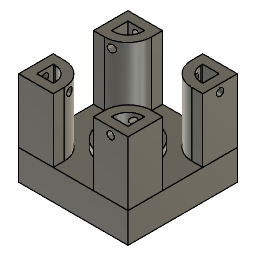
robot (Autodesk Fusion 360 archive; units mm, degrees)
design "pince_v01_structure"
part number: 2026-02-12-14-10-12-234
Autodesk Fusion 360 part; units mm, degrees
(part 1 of 2)
sketch "Esquisse1" plane through (0, 0, 0) normal (0, 0, 1) x (1, 0, 0)
  line L0 (30, 30) -> (-30, 30)
  line L1 (-30, 30) -> (-30, -30)
  line L2 (-30, -30) -> (30, -30)
  line L3 (30, -30) -> (30, 30)
  constraint horizontal L0
  constraint vertical L1
  constraint horizontal L2
  constraint vertical L3
extrude "Extrusion1" add sketch "Esquisse1" along normal blind 5 makes body 1
sketch "Esquisse3" plane through (0, 0, 5) normal (0, 0, 1) x (-1, 0, 0)
  line L0 (-30, 30) -> (-30, -30)
  line L1 (-30, -30) -> (30, -30)
  line L2 (30, -30) -> (30, 30)
  line L3 (30, 30) -> (-30, 30)
  circle A0 centre (0, 0) radius 3.5
  circle A1 centre (0, 0) radius 15
  dimension "d12" = 7
  dimension "d15" = 30
  constraint coincident A0.centre A1.centre
  measures "d12" diameter of A0
  measures "d15" diameter of A1
extrude "Extrusion2" add sketch "Esquisse3" along normal blind 4 contours A1 bodies 1
sketch "Esquisse4" plane through (0, 0, 5) normal (0, 0, 1) x (-1, 0, 0)
  line L0 (-30, 30) -> (-30, -30)
  line L1 (-30, -30) -> (30, -30)
  line L2 (30, -30) -> (30, 30)
  line L3 (30, 30) -> (-30, 30)
  circle A0 centre (0, 0) radius 15
  arc A1 (-24, 11) -> (-11, 24) centre (-24, 24) ccw
  line L4 (-11, 24) -> (-30, 24)
  line L5 (-30, 24) -> (-30, 30)
  line L6 (-30, 30) -> (-11, 30)
  line L7 (-11, 30) -> (-11, 24)
  line L8 (-30, 30) -> (-24, 30)
  line L9 (-24, 30) -> (-24, 11)
  line L10 (-24, 11) -> (-30, 11)
  line L11 (-30, 11) -> (-30, 30)
  constraint horizontal L4
  constraint vertical L5
  constraint horizontal L6
  constraint vertical L7
  constraint coincident L0.start L3.end
  constraint horizontal L8
  constraint vertical L9
  constraint horizontal L10
  constraint vertical L11
extrude "Extrusion3" add sketch "Esquisse4" along normal up to surface (70 mm away) contours L0 L3 L4 L5 L6 L8 L9 L11 | L0 L4 L9 L10 L11 | L3 L4 L6 L7 L9 | A1 L4 L9 bodies 1
sketch "Esquisse5" plane through (0, 0, 0) normal (0, 1, 0) x (1, 0, 0)
  line L0 (-30, 0) -> (30, 0)
  line L1 (30, 0) -> (30, 9.0556)
  line L2 (30, 19.372) -> (-30, 19.372)
  line L3 (-30, 9.0556) -> (-30, 0)
  circle A0 centre (0, 36) radius 34.3
  arc A1 (-25.7143, 10.8052) -> (25.7143, 10.8052) centre (0, 36) ccw
  arc A2 (-25.7143, 10.8052) -> (-30, 9.0556) centre (-27.5, 9.0556) ccw
  arc A3 (30, 9.0556) -> (25.7143, 10.8052) centre (27.5, 9.0556) ccw
  line L4 (-30, 7.5) -> (-27.5, 7.5)
  line L5 (-27.5, 7.5) -> (-27.5, 11.5556)
  line L6 (-27.5, 11.5556) -> (-30, 11.5556)
  line L7 (-30, 11.5556) -> (-30, 7.5)
  point P0 (-30, 0)
  dimension "d80" = 36
  dimension "d81" = 2.5
  dimension "d82" = 2.5
  dimension "d83" = 2.5
  constraint horizontal L0
  constraint vertical L1
  constraint horizontal L2
  constraint vertical L3
  constraint coincident L2.start A0
  constraint coincident P0 L0.start
  constraint coincident A0.centre A1.centre
  constraint tangent A1 A2
  constraint tangent L3 A2
  constraint tangent A1 A3
  constraint tangent L1 A3
  constraint horizontal L4
  constraint vertical L5
  constraint horizontal L6
  constraint vertical L7
  constraint coincident L3 L4.start
  measures "d80" radius of A1
  measures "d81" radius of A2
  measures "d82" radius of A3
  measures "d83" distance of L4.start L4.end
revolve "Révolution2" add sketch "Esquisse5" angle 360 about axis through (0, 0, -205.75) along (0, 0, 1) contours L0 L3 A1 A2 L4 L5 | L3 A2 L4 L5 L7 | A2 L6 L7 bodies 1
extrude "Extrusion4" add 4 faces at (-24.1061, -24.1061, 0) (24.1061, -24.1061, 0) (24.1061, 24.1061, 0) (-24.1061, 24.1061, 0) along direction (0, 0, -1) up to surface end surface through (0, 0, -11.5556) normal (0, 0, -1) offset 0 on bodies 1 bodies 1
extrude "Extrusion5" cut 1 faces at (28, -17.3333, 75) along direction (0, 0, -1) blind 35 on bodies 1 bodies 1
sketch "Esquisse7" plane through (0, 0, 40) normal (0, 0, 1) x (-1, 0, 0)
  line L0 (-30, 11) -> (-24, 11)
  arc A0 (-24, 11) -> (-11, 24) centre (-24, 24) ccw
  line L1 (-11, 24) -> (-11, 30)
  line L2 (-11, 30) -> (-30, 30)
  line L3 (-30, 30) -> (-30, 11)
  line L4 (-16, 24) -> (-16, 25)
  line L5 (-16, 25) -> (-25, 25)
  line L6 (-25, 25) -> (-25, 16)
  line L7 (-25, 16) -> (-24, 16)
  arc A1 (-24, 16) -> (-16, 24) centre (-24, 24) ccw
  dimension "d157" = -5
extrude "Extrusion7" cut sketch "Esquisse7" against normal blind 10 contours L4 L5 L6 L7 A1 bodies 1
pattern_circular "Réseau C2" count 4 over 360 about axis through (0, 0, -205.75) along (0, 0, 1) of bodies 1 makes body 2 at (30, 23.6667, 11.1481) makes body 3 at (-23.6667, 30, 11.1481) makes body 4 at (-30, -23.6667, 11.1481)
sketch "Esquisse8" plane through (0, -30, 0) normal (0, -1, 0) x (1, 0, 0)
  line L0 (30, 40) -> (11, 40)
  line L1 (11, 40) -> (11, 5)
  line L2 (11, 5) -> (-30, 5)
  line L3 (-30, 5) -> (-30, -11.5556)
  line L4 (-30, -11.5556) -> (30, -11.5556)
  line L5 (30, -11.5556) -> (30, 40)
  line L6 (11, 40) -> (30, 40)
  line L7 (30, 40) -> (30, 36)
  line L8 (30, 36) -> (11, 36)
  line L9 (11, 36) -> (11, 40)
  circle A0 centre (20.5, 36) radius 2
  dimension "d3" = 4
  dimension "d4" = 4
  constraint horizontal L6
  constraint vertical L7
  constraint horizontal L8
  constraint vertical L9
  constraint coincident L0.end L1.start
  constraint midpoint L8 A0.centre
  measures "d3" distance of L0.end L8.end
  measures "d4" diameter of A0
extrude "Extrusion8" cut sketch "Esquisse8" against normal up to surface (19 mm away) contours L8 A0 | L8 A0 bodies 1
sketch "Esquisse9" plane through (-30, 0, 0) normal (-1, 0, 0) x (0, -1, 0)
  line L0 (30, 40) -> (11, 40)
  line L1 (11, 40) -> (11, 5)
  line L2 (11, 5) -> (-30, 5)
  line L3 (-30, 5) -> (-30, -11.5556)
  line L4 (-30, -11.5556) -> (30, -11.5556)
  line L5 (30, -11.5556) -> (30, 40)
  line L6 (30, 40) -> (11, 40)
  line L7 (30, 40) -> (30, 36)
  line L8 (30, 36) -> (11, 36)
  line L9 (11, 36) -> (11, 40)
  circle A0 centre (20.5, 36) radius 2
  line L10 (11, 40) -> (30, 40)
  dimension "d7" = 4
  dimension "d8" = 4
  constraint horizontal L10
  constraint vertical L7
  constraint horizontal L8
  constraint vertical L9
  constraint coincident L0.end L1.start
  constraint midpoint A0.centre L8
  measures "d7" distance of L0.end L8.end
  measures "d8" diameter of A0
sketch "Esquisse10" plane through (0, 30, 0) normal (0, 1, 0) x (-1, 0, 0)
  line L0 (30, 40) -> (11, 40)
  line L1 (11, 40) -> (11, 5)
  line L2 (11, 5) -> (-30, 5)
  line L3 (-30, 5) -> (-30, -11.5556)
  line L4 (-30, -11.5556) -> (30, -11.5556)
  line L5 (30, -11.5556) -> (30, 40)
  line L6 (30, 40) -> (11, 40)
  line L7 (30, 40) -> (30, 36)
  line L8 (30, 36) -> (11, 36)
  line L9 (11, 36) -> (11, 40)
  circle A0 centre (20.5, 36) radius 2
  line L10 (11, 40) -> (30, 40)
  dimension "d9" = 4
  dimension "d10" = 4
  constraint horizontal L10
  constraint vertical L7
  constraint horizontal L8
  constraint vertical L9
  constraint coincident L0.end L1.start
  constraint midpoint A0.centre L8
  measures "d9" distance of L0.end L8.end
  measures "d10" diameter of A0
sketch "Esquisse11" plane through (30, 0, 0) normal (1, 0, 0) x (0, 1, 0)
  line L0 (30, 40) -> (11, 40)
  line L1 (11, 40) -> (11, 5)
  line L2 (11, 5) -> (-30, 5)
  line L3 (-30, 5) -> (-30, -11.5556)
  line L4 (-30, -11.5556) -> (30, -11.5556)
  line L5 (30, -11.5556) -> (30, 40)
  line L6 (30, 40) -> (11, 40)
  line L7 (30, 40) -> (30, 36)
  line L8 (30, 36) -> (11, 36)
  line L9 (11, 36) -> (11, 40)
  circle A0 centre (20.5, 36) radius 2
  line L10 (11, 40) -> (30, 40)
  dimension "d11" = 4
  dimension "d16" = 4
  constraint horizontal L10
  constraint vertical L7
  constraint horizontal L8
  constraint vertical L9
  constraint coincident L0.end L1.start
  constraint midpoint A0.centre L8
  measures "d11" distance of L0.end L8.end
  measures "d16" diameter of A0
extrude "Extrusion9" cut sketch "Esquisse9" against normal up to surface (19 mm away) contours L8 A0 | L8 A0 bodies 4
extrude "Extrusion10" cut sketch "Esquisse10" against normal up to surface (19 mm away) contours L8 A0 | L8 A0 bodies 3
extrude "Extrusion11" cut sketch "Esquisse11" against normal up to surface (19 mm away) contours L8 A0 | L8 A0 bodies 2

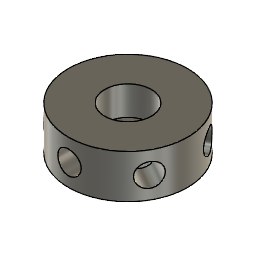
design "encoder_wheel"
part number: 2026-04-24-11-50-52-108
part number: 2026-04-24-11-55-09-590
Autodesk Fusion 360 part; units mm, degrees
sketch "Esquisse1" plane through (0, 0, 0) normal (0, 0, 1) x (1, 0, 0) in component "encoder_wheel"
  line L0 (0, 3.2) -> (-3.2, 0)
  circle A0 centre (0, 0) radius 8.2
  line L1 (-2.5981, -1.5) -> (0, -3)
  line L2 (0, -3) -> (2.5981, -1.5)
  circle A1 centre (0, 0) radius 3.2
  line L3 (-2.5981, 1.5) -> (-2.5981, -1.5)
  line L4 (0, 3) -> (-2.5981, 1.5)
  line L5 (2.5981, -1.5) -> (2.5981, 1.5)
  line L6 (2.5981, 1.5) -> (0, 3)
  dimension "d1" = 6.4
  dimension "d2" = 16.4
  constraint coincident A0.centre A1.centre
  constraint coincident L0.start A1
  constraint coincident L0.end A1
  measures "d1" diameter of A1
  measures "d2" diameter of A0
extrude "Extrusion1" add sketch "Esquisse1" along normal blind 6 in component "encoder_wheel"
extrude "Extrusion2" add sketch "Esquisse1" along normal blind 2 contours L0 A1 L3 L4 | L0 L3 L4 in component "encoder_wheel"
sketch "Esquisse2" plane through (0, 0, 0) normal (0, 1, 0) x (1, 0, 0) in component "encoder_wheel"
  circle A0 through (1.6, -3, -8.2) (-0.8, -1.6144, -8.2) (-0.8, -4.3856, -8.2)
  dimension "d7" = 3.2
extrude "Extrusion3" cut sketch "Esquisse2" along normal blind 3.5 contours A0 in plane through (0, -8.2, 0) normal (0, 1, 0) in component "encoder_wheel"
pattern_circular "Réseau C1" count 6 over 360 about axis through (0, 0, 1.75) along (0, 0, 1) of "Extrusion3" in component "encoder_wheel"
component "encoder_wheel" placed x (1, 0, 0) y (0, 1, 0) z (0, 0, 1) at (0, 0, 0)

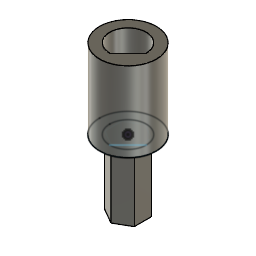
design "wheel-motor_adapter"
part number: 2026-02-08-14-05-17-798
part number: 2026-02-08-22-36-21-611
Autodesk Fusion 360 part; units mm, degrees
sketch "Esquisse1" plane through (0, 0, 0) normal (0, 0, 1) x (1, 0, 0) in component "adaptater"
  line L0 (0, 3) -> (-2.5981, 1.5)
  line L1 (-2.5981, 1.5) -> (-2.5981, -1.5)
  line L2 (-2.5981, -1.5) -> (0, -3)
  line L3 (0, -3) -> (2.5981, -1.5)
  line L4 (2.5981, -1.5) -> (2.5981, 1.5)
  line L5 (2.5981, 1.5) -> (0, 3)
  dimension "d12" = 3
  measures "d12" distance of L0.start origin
extrude "Extrusion1" add sketch "Esquisse1" along normal blind 12 makes body 1 in component "adaptater"
sketch "Esquisse2" plane through (0, 0, 12) normal (0, 0, 1) x (-1, 0, 0) in component "adaptater"
  line L0 (-2.5981, -1.5) -> (0, -3)
  line L1 (0, -3) -> (2.5981, -1.5)
  line L2 (2.5981, -1.5) -> (2.5981, 1.5)
  line L3 (2.5981, 1.5) -> (0, 3)
  line L4 (0, 3) -> (-2.5981, 1.5)
  line L5 (-2.5981, 1.5) -> (-2.5981, -1.5)
  circle A0 centre (0, 0) radius 3.2
  circle A1 centre (0, 0) radius 5
  line L6 (0, 3.2) -> (-3.2, 0)
  dimension "d15" = 6.4
  dimension "d16" = 10
  constraint coincident A0.centre A1.centre
  constraint coincident A0 L6.start
  constraint coincident A0 L6.end
  measures "d15" diameter of A0
  measures "d16" diameter of A1
extrude "Extrusion2" add sketch "Esquisse2" along normal blind 14 bodies 1 makes body 2 in component "adaptater"
extrude "Extrusion3" add sketch "Esquisse2" along normal blind 4 contours L0 L1 L2 L3 L4 L5 L6 | L0 L1 L2 L3 L4 L5 A0 L6 | L4 L5 L6 bodies 1 2 in component "adaptater"
extrude "Extrusion4" add sketch "Esquisse2" along normal blind 4 contours L4 L5 A0 L6 bodies 1 in component "adaptater"
extrude "Extrusion5" add sketch "Esquisse2" along normal blind 14 contours L4 L5 A0 L6 | L4 L5 L6 bodies 1 in component "adaptater"
component "adaptater" placed x (1, 0, 0) y (0, 1, 0) z (0, 0, 1) at (0, 0, 0)

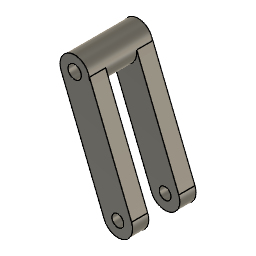
design "pince_v01_second_arm"
part number: 2026-02-12-19-33-38-702
Autodesk Fusion 360 part; units mm, degrees
sketch "Esquisse1" plane through (0, -10.5, 0) normal (0, 1, 0) x (-1, 0, 0)
  circle A0 centre (-25, 50) radius 2
  line L0 (-30, 56) -> (-30, 40)
  line L1 (-30, 40) -> (-18, 40)
  line L2 (-18, 40) -> (-18, 56)
  line L3 (-18, 56) -> (-30, 56)
  circle A1 centre (-25, 50) radius 2.25
  circle A2 centre (-25, 50) radius 5
  circle A3 centre (-39.6076, 13.6901) radius 5
  circle A4 centre (-39.6076, 13.6901) radius 2
  line L4 (-25, 50) -> (-39.6076, 13.6901)
  line L5 (-29.6387, 51.8662) -> (-44.2463, 15.5563)
  line L6 (-20.3613, 48.1338) -> (-34.9689, 11.824)
  point P0 (-22.75, 50.0115)
  point P1 (-39.6076, 13.6901)
  dimension "d228" = 10
  dimension "d229" = 10
  dimension "d230" = 4
  constraint concentric A0 A1
  constraint coincident A1 P0
  constraint concentric A1 A2
  constraint coincident P1 A3.centre
  constraint concentric A3 A4
  constraint coincident A0.centre A1.centre
  measures "d228" diameter of A2
  measures "d229" diameter of A3
  measures "d230" diameter of A4
extrude "Extrusion1" add sketch "Esquisse1" along normal blind 5.25 contours L0 L1 A3 L4 L5 | L0 L1 A2 L4 | A3 | L1 A2 L4 L6 | L1 A3 L4 L6
extrude "Extrusion2" add sketch "Esquisse1" along normal blind 10.5 contours A2
move_body "Déplacer1" bodies 1 to x (1, 0, 0) y (0, 1, 0) z (0, 0, 1) at (0, 0.25, 0)
extrude "Extrusion3" cut 1 faces at (31.7625, -10.25, 37.8971) along direction (0, 1, 0) blind 0.25
extrude "Extrusion4" cut 1 faces at (20.9437, 0.25, 50.3602) along direction (0, -1, 0) blind 0.25
mirror "Symétrie miroir1" about plane through (0, 0, 0) normal (0, 1, 0) of bodies 1 merged
extrude "Extrusion5" add 1 faces at (31.7625, -10, 37.8971) along direction (0, -1, 0) blind 0.25
extrude "Extrusion6" cut 1 faces at (37.5808, -5, 25.9737) along direction (0, -1, 0) blind 0.25
extrude "Extrusion7" add 1 faces at (31.7625, 10, 37.8971) along direction (0, 1, 0) blind 0.25
extrude "Extrusion8" cut 1 faces at (37.5808, 5, 25.9737) along direction (0, 1, 0) blind 0.25
extrude "Extrusion9" add 1 faces at (31.7625, -10.25, 37.8971) along direction (0, -1, 0) blind 0.5
extrude "Extrusion10" add 1 faces at (31.7625, 10.25, 37.8971) along direction (0, 1, 0) blind 0.5

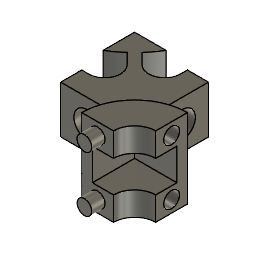
design "pince"
part number: 2026-02-08-14-04-40-905
part number: 2026-02-09-15-39-11-388
part number: 2026-02-09-16-45-21-532
Autodesk Fusion 360 part; units mm, degrees
sketch "Esquisse1" plane through (0, 0, 0) normal (0, 0, 1) x (1, 0, 0) in component "structure"
  line L0 (0, 0) -> (30, 0)
  line L1 (30, 0) -> (30, 30)
  line L2 (30, 30) -> (0, 30)
  line L3 (0, 30) -> (0, 0)
  line L4 (30, 30) -> (-30, 30)
  line L5 (-30, 30) -> (-30, -30)
  line L6 (-30, -30) -> (30, -30)
  line L7 (30, -30) -> (30, 30)
  line L8 (-30, 30) -> (-10, 30)
  line L9 (-10, 30) -> (-10, 10)
  line L10 (-10, 10) -> (-30, 10)
  line L11 (-30, 10) -> (-30, 30)
  circle A0 centre (-30, 30) radius 20
  circle A1 centre (-30, 30) radius 18
  line L12 (-30, 30) -> (-5, 10)
  line L13 (-30, 30) -> (-10, 5)
  line L14 (-10, 10) -> (-22, 10)
  line L15 (-22, 10) -> (-22, 22)
  line L16 (-22, 22) -> (-10, 22)
  line L17 (-10, 22) -> (-10, 10)
  dimension "d1" = 30
  dimension "d2" = 30
  dimension "d3" = 60
  dimension "d4" = 60
  dimension "d5" = 12
  dimension "d6" = 12
  constraint horizontal L0
  constraint vertical L1
  constraint horizontal L2
  constraint vertical L3
  constraint coincident L0.start L3.end
  constraint horizontal L4
  constraint vertical L5
  constraint horizontal L6
  constraint vertical L7
  constraint horizontal L8
  constraint vertical L9
  constraint horizontal L10
  constraint vertical L11
  constraint coincident L4.end L5.start
  constraint coincident L8.end A0
  constraint concentric A0 A1
  constraint horizontal L14
  constraint vertical L15
  constraint horizontal L16
  constraint vertical L17
  measures "d1" distance of L0.start L0.end
  measures "d2" distance of L0.start L2.end
  measures "d3" distance of L1.end L4.end
  measures "d4" distance of L1.end L6.end
  measures "d5" distance of L9.end L14.end
  measures "d6" distance of L9.end L16.end
extrude "Extrusion1" add sketch "Esquisse1" along normal blind 60 contours L4 L8 A0 A1 L16 | L4 L8 A1 L12 L16 | L5 L11 A0 A1 L15 | A0 A1 L12 L16 | L5 L11 A1 L13 L15 | L12 L13 L15 L16 | A0 A1 L13 L15 makes body 1 in component "structure"
pattern_circular "Réseau C1" count 4 over 360 about axis through (0, 0, 1.75) along (0, 0, 1) of bodies 1 makes body 2 at (-30, -18, 20) makes body 3 at (18, -30, 20) makes body 4 at (30, 18, 20) in component "structure"
extrude "Extrusion2" add sketch "Esquisse1" along normal blind 10 contours L0 L1 L2 L3 L4 L7 | L0 L3 L4 L5 L6 L7 L9 L10 L14 L17 | L4 L8 A0 A1 L16 | L9 A0 L16 | L4 L8 A1 L12 L16 | L9 A0 L12 L16 L17 | L10 A0 L15 | L5 L11 A0 A1 L15 | A0 A1 L12 L16 | L5 L11 A1 L13 L15 | L12 L13 L15 L16 | A1 L12 L16 | L9 L10 A0 L12 L13 L14 L17 | L10 A0 L13 L14 L15 | A0 A1 L13 L15 | A0 A1 L12 L13 | A1 L12 L13 L15 L16 | A1 L13 L15 bodies 1 2 3 4 in component "structure"
sketch "Esquisse1 (2)" plane through (0, 0, 10) normal (0, 0, 1) x (-1, 0, 0) in component "mobile"
  arc A0 (-14.3826, 17.5061) -> (-10, 30) centre (-30, 30) ccw
  line L0 (-14.3826, 17.5061) -> (-15.9444, 18.7555)
  arc A1 (-15.9444, 18.7555) -> (-13.8755, 22) centre (-30, 30) ccw
  line L1 (-13.8755, 22) -> (-22, 22)
  line L2 (-22, 22) -> (-22, 13.8755)
  arc A2 (-22, 13.8755) -> (-18.7555, 15.9444) centre (-30, 30) ccw
  line L3 (-18.7555, 15.9444) -> (-17.5061, 14.3826)
  arc A3 (-30, 10) -> (-17.5061, 14.3826) centre (-30, 30) ccw
  line L4 (-30, 10) -> (-30, -10)
  arc A4 (-17.5061, -14.3826) -> (-30, -10) centre (-30, -30) ccw
  line L5 (-17.5061, -14.3826) -> (-18.7555, -15.9444)
  arc A5 (-18.7555, -15.9444) -> (-22, -13.8755) centre (-30, -30) ccw
  line L6 (-22, -13.8755) -> (-22, -22)
  line L7 (-22, -22) -> (-13.8755, -22)
  arc A6 (-13.8755, -22) -> (-15.9444, -18.7555) centre (-30, -30) ccw
  line L8 (-15.9444, -18.7555) -> (-14.3826, -17.5061)
  arc A7 (-10, -30) -> (-14.3826, -17.5061) centre (-30, -30) ccw
  line L9 (-10, -30) -> (10, -30)
  arc A8 (14.3826, -17.5061) -> (10, -30) centre (30, -30) ccw
  line L10 (14.3826, -17.5061) -> (15.9444, -18.7555)
  arc A9 (15.9444, -18.7555) -> (13.8755, -22) centre (30, -30) ccw
  line L11 (13.8755, -22) -> (22, -22)
  line L12 (22, -22) -> (22, -13.8755)
  arc A10 (22, -13.8755) -> (18.7555, -15.9444) centre (30, -30) ccw
  line L13 (18.7555, -15.9444) -> (17.5061, -14.3826)
  arc A11 (30, -10) -> (17.5061, -14.3826) centre (30, -30) ccw
  line L14 (30, -10) -> (30, 10)
  arc A12 (17.5061, 14.3826) -> (30, 10) centre (30, 30) ccw
  line L15 (17.5061, 14.3826) -> (18.7555, 15.9444)
  arc A13 (18.7555, 15.9444) -> (22, 13.8755) centre (30, 30) ccw
  line L16 (22, 13.8755) -> (22, 22)
  line L17 (22, 22) -> (13.8755, 22)
  arc A14 (13.8755, 22) -> (15.9444, 18.7555) centre (30, 30) ccw
  line L18 (15.9444, 18.7555) -> (14.3826, 17.5061)
  arc A15 (10, 30) -> (14.3826, 17.5061) centre (30, 30) ccw
  line L19 (10, 30) -> (-10, 30)
  arc A16 (22, -13.8755) -> (13.8755, -22) centre (30, -30) ccw
  line L20 (22, -13.8755) -> (22, -22)
  line L21 (13.8755, -22) -> (22, -22)
  line L22 (21.2, -15.2216) -> (21.2, -21.2)
  line L23 (15.2216, -21.2) -> (21.2, -21.2)
  arc A17 (21.2, -15.2216) -> (15.2216, -21.2) centre (30, -30) ccw
  line L24 (0, 0) -> (17.8378, -17.8378)
  line L25 (0, 0) -> (25.2264, 0) construction
  line L26 (8.2929, -9.7071) -> (17.1307, -18.5449)
  arc A18 (0, -10) -> (4.3096, -9.0237) centre (0, 0) ccw
  line L27 (10, 0) -> (0, 0)
  line L28 (0, -10) -> (0, 0)
  line L29 (18.5449, -17.1307) -> (18.5654, -17.1512)
  line L30 (17.1307, -18.5449) -> (17.1512, -18.5654)
  arc A19 (8.2929, -9.7071) -> (4.3096, -9.0237) centre (5.818, -12.182) ccw
  line L31 (10, 0) -> (0, 0)
  arc A20 (9.0237, -4.3096) -> (10, 0) centre (0, 0) ccw
  arc A21 (9.0237, -4.3096) -> (9.7071, -8.2929) centre (12.182, -5.818) ccw
  line L32 (9.7071, -8.2929) -> (18.5449, -17.1307)
  line L33 (18.5449, -17.1307) -> (18.5654, -17.1512)
  dimension "d13" = 0.8
  dimension "d14" = 45
  dimension "d17" = 3.5
  constraint coincident L12.end A10.start
  constraint coincident A9.end L11.start
  constraint coincident L11.end L12.start
  constraint horizontal L25
  constraint coincident L24.start L25.start
  constraint coincident A17 L24.end
  constraint coincident L25 L27.start
  constraint perpendicular L27 L28
  constraint coincident A17 L29.end
  constraint coincident A17 L30.end
  constraint parallel L26 L30
  constraint tangent A18 A19
  constraint tangent L26 A19
  constraint symmetric L24 L26.end L29.start
  constraint symmetric L24 A18.start L27.start
  constraint symmetric L24 A18 A20
  constraint symmetric L24 L25.start A18.centre
  constraint symmetric L24 L30.end L29.end
  constraint symmetric L24 L26.start A21.end
  constraint symmetric L24 A18.end A20.start
  constraint symmetric L24 A19 A21
  measures "d14" angle of L24 L25
  measures "d17" radius of A19
extrude "Extrusion1'" add sketch "Esquisse1 (2)" along normal blind 10 separate body contours A16 A17 L24 L29 L32 L33 | A16 L24 L27 L31 A20 A21 L32 | A16 A17 L24 L26 L30 | A16 L24 L26 A18 L28 A19 | L22 L23 A17 makes body 5 in component "mobile"
sketch "Esquisse2" plane through (0, 0, 20) normal (0, 0, 1) x (-1, 0, 0) in component "mobile"
  arc A0 (9.0237, -4.3096) -> (10, 0) centre (0, 0) ccw
  line L0 (10, 0) -> (0, 0)
  line L1 (0, 0) -> (0, -10)
  arc A1 (0, -10) -> (4.3096, -9.0237) centre (0, 0) ccw
  arc A2 (8.2929, -9.7071) -> (4.3096, -9.0237) centre (5.818, -12.182) ccw
  line L2 (8.2929, -9.7071) -> (17.1512, -18.5654)
  arc A3 (17.1512, -18.5654) -> (15.2216, -21.2) centre (30, -30) ccw
  line L3 (15.2216, -21.2) -> (21.2, -21.2)
  line L4 (21.2, -21.2) -> (21.2, -15.2216)
  arc A4 (21.2, -15.2216) -> (18.5654, -17.1512) centre (30, -30) ccw
  line L5 (18.5654, -17.1512) -> (9.7071, -8.2929)
  arc A5 (9.0237, -4.3096) -> (9.7071, -8.2929) centre (12.182, -5.818) ccw
  arc A6 (0, -10) -> (10, 0) centre (0, 0) ccw
  constraint coincident L1.end A1.start
  constraint coincident A0.end L0.start
extrude "Extrusion2'" add sketch "Esquisse2" along normal blind 5 contours A0 L0 L1 A1 A6 bodies 5 in component "mobile"
sketch "Esquisse3" plane through (0, 0, 10) normal (0, 0, -1) x (1, 0, 0) in component "mobile"
  arc A0 (-10, 0) -> (-9.0237, -4.3096) centre (0, 0) ccw
  arc A1 (-9.7071, -8.2929) -> (-9.0237, -4.3096) centre (-12.182, -5.818) ccw
  line L0 (-9.7071, -8.2929) -> (-18.5654, -17.1512)
  arc A2 (-18.5654, -17.1512) -> (-21.2, -15.2216) centre (-30, -30) ccw
  line L1 (-21.2, -15.2216) -> (-21.2, -21.2)
  line L2 (-21.2, -21.2) -> (-15.2216, -21.2)
  arc A3 (-15.2216, -21.2) -> (-17.1512, -18.5654) centre (-30, -30) ccw
  line L3 (-17.1512, -18.5654) -> (-8.2929, -9.7071)
  arc A4 (-4.3096, -9.0237) -> (-8.2929, -9.7071) centre (-5.818, -12.182) ccw
  arc A5 (-4.3096, -9.0237) -> (0, -10) centre (0, 0) ccw
  line L4 (0, -10) -> (0, 0)
  line L5 (0, 0) -> (-10, 0)
  arc A6 (-10, 0) -> (0, -10) centre (0, 0) ccw
  constraint coincident A0.start L5.end
  constraint coincident A5.end L4.start
extrude "Extrusion3" cut sketch "Esquisse3" against normal blind 5 contours A1 L0 A2 L1 L2 A3 L3 A4 A6 bodies 5 in component "mobile"
sketch "Esquisse4" plane through (0, 0, 0) normal (1, 0, 0) x (0, 1, 0) in component "mobile"
  line L0 (0, 10) -> (10, 10)
  line L1 (10, 10) -> (10, 25)
  line L2 (10, 25) -> (0, 25)
  line L3 (0, 25) -> (0, 10)
  line L4 (5, 25) -> (5, 22.5)
  circle A0 centre (5, 22.5) radius 1.25
  line L5 (5, 10) -> (5, 12.5)
  circle A1 centre (5, 12.5) radius 1.25
  dimension "d24" = 2.5
  dimension "d25" = 2.5
  dimension "d26" = 2.5
  dimension "d27" = 2.5
  constraint midpoint L2 L4.start
  constraint perpendicular L2 L4
  constraint coincident L4.end A0.centre
  constraint midpoint L0 L5.start
  constraint perpendicular L0 L5
  constraint coincident L5.end A1.centre
  measures "d24" distance of L4.start L4.end
  measures "d25" diameter of A0
  measures "d26" distance of L5.start L5.end
  measures "d27" diameter of A1
extrude "Extrusion4" cut sketch "Esquisse4" against normal blind 4 contours A0 | A1 bodies 5 in component "mobile"
sketch "Esquisse5" plane through (0, 0, 0) normal (0, -1, 0) x (1, 0, 0) in component "mobile"
  line L0 (-10, 10) -> (0, 10)
  line L1 (0, 10) -> (0, 25)
  line L2 (0, 25) -> (-10, 25)
  line L3 (-10, 25) -> (-10, 10)
  line L4 (-5, 25) -> (-5, 22.5)
  circle A0 centre (-5, 22.5) radius 1
  line L5 (-5, 10) -> (-5, 12.5)
  circle A1 centre (-5, 12.5) radius 1
  dimension "d30" = 2.5
  dimension "d31" = 2
  dimension "d32" = 2.5
  dimension "d33" = 2
  constraint midpoint L2 L4.start
  constraint perpendicular L2 L4
  constraint coincident L4.end A0.centre
  constraint midpoint L0 L5.start
  constraint perpendicular L0 L5
  constraint coincident L5.end A1.centre
  measures "d30" distance of L4.start L4.end
  measures "d31" diameter of A0
  measures "d32" distance of L5.start L5.end
  measures "d33" diameter of A1
extrude "Extrusion5" add sketch "Esquisse5" along normal blind 3.5 contours A0 | A1 bodies 5 in component "mobile"
sketch "Esquisse6" plane through (0, 0, 0) normal (1, 0, 0) x (0, 1, 0) in component "mobile"
  circle A0 centre (5, 22.5) radius 1.25
  circle A1 centre (5, 12.5) radius 1.25
  line L0 (0, 10) -> (10, 10)
  line L1 (10, 10) -> (10, 25)
  line L2 (10, 25) -> (0, 25)
  line L3 (0, 25) -> (0, 10)
  line L4 (9, 10) -> (20, 10)
  line L5 (20, 10) -> (20, 25)
  line L6 (20, 25) -> (9, 25)
  line L7 (9, 25) -> (9, 10)
  dimension "d36" = 11
  dimension "d37" = 15
  constraint horizontal L4
  constraint vertical L5
  constraint horizontal L6
  constraint vertical L7
  constraint coincident L0 L4.start
  measures "d36" distance of L4.start L4.end
  measures "d37" distance of L4.start L6.end
extrude "Extrusion6" add sketch "Esquisse6" against normal blind 10 contours L0 L1 L2 L4 L6 L7 | L1 L4 L5 L6 bodies 5 in component "mobile"
extrude "Extrusion7" add 1 faces at (-7.2116, 9, 23.3333) along direction (0, -1, 0) up to surface (9 mm away) on bodies 5 bodies 5 in component "mobile"
extrude "Extrusion8" cut sketch "Esquisse6" against normal blind 6 contours L1 L4 L5 L6 bodies 5 in component "mobile"
sketch "Esquisse7" plane through (-6, 0, 0) normal (1, 0, 0) x (0, 1, 0) in component "mobile"
  line L0 (10, 10) -> (20, 10)
  line L1 (20, 10) -> (20, 25)
  line L2 (20, 25) -> (10, 25)
  line L3 (10, 25) -> (10, 10)
  circle A0 centre (15, 17.5) radius 2.5
  dimension "d44" = 5
  measures "d44" diameter of A0
extrude "Extrusion9" cut sketch "Esquisse7" against normal up to surface (4 mm away) contours A0 bodies 5 in component "mobile"
sketch "Esquisse8" plane through (0, 0, 0) normal (0, -1, 0) x (1, 0, 0) in component "mobile"
  line L0 (-10, 10) -> (0, 10)
  line L1 (0, 10) -> (0, 25)
  line L2 (0, 25) -> (-10, 25)
  line L3 (-10, 25) -> (-10, 20)
  line L4 (-10, 20) -> (-10, 15)
  line L5 (-10, 15) -> (-10, 10)
  circle A0 centre (-5, 12.5) radius 1
  circle A1 centre (-5, 22.5) radius 1
  line L6 (-7, 25) -> (-20, 25)
  line L7 (-20, 25) -> (-20, 10)
  line L8 (-20, 10) -> (-7, 10)
  line L9 (-7, 10) -> (-7, 25)
  dimension "d47" = 13
  dimension "d48" = 15
  constraint horizontal L6
  constraint vertical L7
  constraint horizontal L8
  constraint vertical L9
  constraint coincident L2 L6.start
  measures "d47" distance of L6.start L6.end
  measures "d48" distance of L6.start L8.end
extrude "Extrusion10" add sketch "Esquisse8" against normal blind 10 contours L0 L2 L3 L4 L5 L6 L8 L9 | L3 L4 L5 L6 L7 L8 bodies 5 in component "mobile"
extrude "Extrusion11" cut sketch "Esquisse8" against normal blind 5 contours L3 L4 L5 L6 L7 L8 bodies 5 in component "mobile"
sketch "Esquisse9" plane through (0, 5, 0) normal (0, -1, 0) x (1, 0, 0) in component "mobile"
  line L0 (-10, 25) -> (-20, 25)
  line L1 (-20, 25) -> (-20, 10)
  line L2 (-20, 10) -> (-10, 10)
  line L3 (-10, 10) -> (-10, 15)
  line L4 (-10, 15) -> (-10, 20)
  line L5 (-10, 20) -> (-10, 25)
  circle A0 centre (-15, 17.5) radius 2.5
  dimension "d53" = 5
  measures "d53" diameter of A0
extrude "Extrusion12" cut sketch "Esquisse9" against normal blind 5 contours A0 bodies 5 in component "mobile"
extrude "Extrusion13" cut 1 faces at (-14.9377, 5, 11.669) along direction (0, 1, 0) blind 1 on bodies 5 bodies 5 in component "mobile"
sketch "Esquisse10" plane through (0, 0, 25) normal (0, 0, 1) x (-1, 0, 0) in component "mobile"
  line L0 (20, -6) -> (10, -6)
  line L1 (10, -6) -> (10, 0)
  line L2 (10, 0) -> (0, 0)
  line L3 (0, 0) -> (0, -10)
  line L4 (0, -10) -> (6, -10)
  line L5 (6, -10) -> (6, -20)
  line L6 (6, -20) -> (10, -20)
  line L7 (10, -20) -> (10, -10)
  line L8 (10, -10) -> (20, -10)
  line L9 (20, -10) -> (20, -6)
  arc A0 (0, -10) -> (10, 0) centre (0, 0) ccw
  constraint coincident L3.end L4.start
  constraint coincident L1.end L2.start
extrude "Extrusion14" cut sketch "Esquisse10" against normal blind 3 contours L0 L1 L4 L5 L6 L7 L8 L9 A0 bodies 5 in component "mobile"
sketch "Esquisse11" plane through (0, 0, 10) normal (0, 0, -1) x (1, 0, 0) in component "mobile"
  line L0 (-10, 0) -> (-10, -6)
  line L1 (-10, -6) -> (-20, -6)
  line L2 (-20, -6) -> (-20, -10)
  line L3 (-20, -10) -> (-10, -10)
  line L4 (-10, -10) -> (-10, -20)
  line L5 (-10, -20) -> (-6, -20)
  line L6 (-6, -20) -> (-6, -10)
  line L7 (-6, -10) -> (0, -10)
  line L8 (0, -10) -> (0, 0)
  line L9 (0, 0) -> (-10, 0)
  arc A0 (-10, 0) -> (0, -10) centre (0, 0) ccw
  constraint coincident L7.end L8.start
  constraint coincident L0.start L9.end
extrude "Extrusion15" cut sketch "Esquisse11" against normal blind 3 contours L0 L1 L2 L3 L4 L5 L6 L7 A0 bodies 5 in component "mobile"
sketch "Esquisse12" plane through (0, 0, 0) normal (1, 0, 0) x (0, 1, 0) in component "mobile"
  line L0 (10, 10) -> (10, 13)
  line L1 (10, 13) -> (10, 22)
  line L2 (10, 22) -> (10, 25)
  line L3 (10, 25) -> (0, 25)
  line L4 (0, 25) -> (0, 10)
  line L5 (0, 10) -> (10, 10)
  circle A0 centre (5, 12.5) radius 1.25
  circle A1 centre (5, 22.5) radius 1.25
  line L6 (0, 17.5) -> (8, 17.5)
  line L7 (8, 17.5) -> (8, 20.5)
  line L8 (8, 20.5) -> (0, 20.5)
  line L9 (0, 20.5) -> (0, 17.5)
  line L10 (8, 14.5) -> (0, 14.5)
  line L11 (0, 14.5) -> (0, 17.5)
  line L12 (8, 17.5) -> (8, 14.5)
  line L13 (0, 17.5) -> (8, 17.5)
  dimension "d64" = 8
  dimension "d65" = 3
  constraint horizontal L6
  constraint vertical L7
  constraint horizontal L8
  constraint vertical L9
  constraint midpoint L4 L6.start
  constraint symmetric L9.end L6 L11.end
  constraint symmetric L7.start L6 L12.start
  constraint symmetric L7.end L6 L10.start
  constraint symmetric L8.end L6 L10.end
  measures "d64" distance of L6.start L6.end
  measures "d65" distance of L6.start L8.end
extrude "Extrusion16" cut sketch "Esquisse12" against normal blind 8 contours L4 L6 L10 L11 L12 L13 | L4 L6 L7 L8 L9 L13 bodies 5 in component "mobile"
sketch "Esquisse13" plane through (0, 0, 25) normal (0, 0, 1) x (-1, 0, 0) in component "mobile"
  arc A0 (0, -10) -> (10, 0) centre (0, 0) ccw
  line L0 (10, 0) -> (0, 0)
  line L1 (0, 0) -> (0, -10)
  circle A1 centre (0, 0) radius 4
  constraint concentric A0 A1
extrude "Extrusion17" cut 2 faces at (-4.7246, -3.5, 22.3122) (-5.1594, -3.5, 13.1014) along direction (0, -1, 0) up to surface end surface through (-10, 0, 10) normal (0, -1, 0) offset 0 on bodies 5 bodies 5 in component "mobile"
extrude "Extrusion18" add 2 faces at (-4, 5.3754, 22.3192) (-4, 5.3443, 12.8589) along direction (1, 0, 0) blind 4 on bodies 5 bodies 5 in component "mobile"
extrude "Extrusion19" cut sketch "Esquisse13" against normal blind 15 contours L0 L1 A1 picked at (0.1898, -2.6531) bodies 5 in component "mobile"
sketch "Esquisse14" plane through (0, 0, 0) normal (1, 0, 0) x (0, 1, 0) in component "mobile"
  line L0 (4, 14.5) -> (4, 10)
  line L1 (4, 10) -> (10, 10)
  line L2 (10, 10) -> (10, 13)
  line L3 (10, 13) -> (10, 22)
  line L4 (10, 22) -> (10, 25)
  line L5 (10, 25) -> (4, 25)
  line L6 (4, 25) -> (4, 20.5)
  line L7 (4, 20.5) -> (8, 20.5)
  line L8 (8, 20.5) -> (8, 14.5)
  line L9 (8, 14.5) -> (4, 14.5)
  line L10 (4, 22.75) -> (10, 22.75)
  circle A0 centre (7, 22.75) radius 1.5
  circle A1 centre (7, 12.25) radius 1.5
  dimension "d74" = 3
  dimension "d75" = 3
  constraint midpoint L6 L10.start
  constraint coincident L4 L10.end
  constraint perpendicular L4 L10
  constraint midpoint L10 A0.centre
  measures "d74" diameter of A0
  measures "d75" diameter of A1
extrude "Extrusion20" cut sketch "Esquisse14" against normal blind 3 contours L10 A0 | L10 A0 | A1 bodies 5 in component "mobile"
sketch "Esquisse15" plane through (0, 0, 0) normal (0, -1, 0) x (1, 0, 0) in component "mobile"
  line L0 (-4, 10) -> (-4, 14.5)
  line L1 (-4, 14.5) -> (-8, 14.5)
  line L2 (-8, 14.5) -> (-8, 20.5)
  line L3 (-8, 20.5) -> (-4, 20.5)
  line L4 (-4, 20.5) -> (-4, 25)
  line L5 (-4, 25) -> (-10, 25)
  line L6 (-10, 25) -> (-10, 22)
  line L7 (-10, 22) -> (-10, 20)
  line L8 (-10, 20) -> (-10, 15)
  line L9 (-10, 15) -> (-10, 13)
  line L10 (-10, 13) -> (-10, 10)
  line L11 (-10, 10) -> (-4, 10)
  circle A0 centre (-7, 22.75) radius 1.4
  circle A1 centre (-7, 12.25) radius 1.4
  dimension "d78" = 2.8
  dimension "d79" = 2.8
  measures "d78" diameter of A0
  measures "d79" diameter of A1
extrude "Extrusion21" add sketch "Esquisse15" along normal blind 2.5 contours A0 | A1 bodies 5 in component "mobile"
extrude "Extrusion22" add 1 faces at (-15.2389, 15.7103, 20) along direction (0, 0, 1) blind 2 on bodies 5 bodies 5 in component "mobile"
extrude "Extrusion23" add 1 faces at (-15.2389, 15.7103, 15) along direction (0, 0, -1) blind 2 on bodies 5 bodies 5 in component "mobile"
sketch "Esquisse16" plane through (0, 0, 22) normal (0, 0, 1) x (-1, 0, 0) in component "mobile"
  line L0 (6, -10) -> (6, -20)
  line L1 (6, -20) -> (10, -20)
  line L2 (10, -20) -> (10, -11.4142)
  line L3 (10, -11.4142) -> (17.1512, -18.5654)
  arc A0 (17.1512, -18.5654) -> (15.2216, -21.2) centre (30, -30) ccw
  line L4 (15.2216, -21.2) -> (21.2, -21.2)
  line L5 (21.2, -21.2) -> (21.2, -15.2216)
  arc A1 (21.2, -15.2216) -> (18.5654, -17.1512) centre (30, -30) ccw
  line L6 (18.5654, -17.1512) -> (11.4142, -10)
  line L7 (11.4142, -10) -> (20, -10)
  line L8 (20, -10) -> (20, -6)
  line L9 (20, -6) -> (10, -6)
  line L10 (10, -6) -> (10, 0)
  arc A2 (0, -10) -> (10, 0) centre (0, 0) ccw
  line L11 (0, -10) -> (6, -10)
  line L12 (10, -20) -> (10, -18.6569)
  line L13 (15.1213, -16.5355) -> (17.1512, -18.5654)
  arc A3 (15.1213, -16.5355) -> (10, -18.6569) centre (13, -18.6569) ccw
  line L14 (18.5654, -17.1512) -> (16.5355, -15.1213)
  line L15 (20, -10) -> (18.6569, -10)
  arc A4 (18.6569, -10) -> (16.5355, -15.1213) centre (18.6569, -13) ccw
  dimension "d86" = 3
  dimension "d87" = 3
  constraint coincident L1.end L2.start
  constraint coincident L3.end A0.start
  constraint tangent L12 A3
  constraint tangent L13 A3
  constraint coincident A1.end L6.start
  constraint coincident L7.end L8.start
  constraint tangent L14 A4
  constraint tangent L15 A4
  measures "d86" radius of A3
  measures "d87" radius of A4
extrude "Extrusion24" add sketch "Esquisse16" against normal blind 9 contours L2 L3 A3 | L6 L7 A4 bodies 5 in component "mobile"
component "structure" placed x (1, 0, 0) y (0, 1, 0) z (0, 0, 1) at (0, 0, 0)
component "mobile" placed x (1, 0, 0) y (0, 1, 0) z (0, 0, 1) at (0, 0, 0)

design "FPGA"
part number: 2026-04-30-13-27-36-560
Autodesk Fusion 360 part; units mm, degrees
sketch "Esquisse1" plane through (0, 0, 0) normal (0, 1, 0) x (1, 0, 0)
  line L0 (-25, 25) -> (55, 25)
  line L1 (55, 25) -> (55, -74)
  line L2 (55, -74) -> (-25, -74)
  line L3 (-25, -74) -> (-25, 25)
  line L4 (-25, 25) -> (-15, 25)
  line L5 (-15, 25) -> (14, 25)
  line L6 (14, 25) -> (14, 33)
  line L7 (14, 33) -> (-15, 33)
  line L8 (-15, 33) -> (-15, 25)
  line L9 (-25, -74) -> (-6, -74)
  line L10 (-6, -74) -> (7, -74)
  line L11 (7, -74) -> (7, -77)
  line L12 (7, -77) -> (-6, -77)
  line L13 (-6, -77) -> (-6, -74)
  dimension "d1" = 80
  dimension "d2" = 99
  dimension "d3" = 10
  dimension "d4" = 29
  dimension "d5" = 8
  dimension "d6" = 19
  dimension "d7" = 13
  dimension "d8" = 3
  constraint horizontal L0
  constraint vertical L1
  constraint horizontal L2
  constraint vertical L3
  constraint perpendicular L3 L4
  constraint horizontal L5
  constraint vertical L6
  constraint horizontal L7
  constraint vertical L8
  constraint perpendicular L3 L9
  constraint horizontal L10
  constraint vertical L11
  constraint horizontal L12
  constraint vertical L13
  measures "d1" distance of L0.start L0.end
  measures "d2" distance of L0.start L2.end
  measures "d3" distance of L0.start L4.end
  measures "d4" distance of L4.end L5.end
  measures "d5" distance of L4.end L7.end
  measures "d6" distance of L2.end L9.end
  measures "d7" distance of L9.end L10.end
  measures "d8" distance of L9.end L12.end
extrude "Extrusion1" add sketch "Esquisse1" along normal blind 20 contours L0 L1 L2 L3 L4 L5 L9 L10
extrude "Extrusion2" add sketch "Esquisse1" along normal blind 20 contours L0 L5 L6 L7 L8
extrude "Extrusion3" add sketch "Esquisse1" along normal blind 20 contours L2 L10 L11 L12 L13

design "pince_v02_mobile"
part number: 2026-02-11-00-55-34-916
Autodesk Fusion 360 part; units mm, degrees
sketch "Esquisse1" plane through (0, 0, 5) normal (0, 0, 1) x (-1, 0, 0)
  line L0 (0, 0, 20) -> (-15, 0, 20)
  line L1 (-15, 0, 20) -> (-15, 15, 20)
  line L2 (-15, 15, 20) -> (0, 15, 20)
  line L3 (0, 15, 20) -> (0, 0, 20)
  dimension "d16" = 15
  dimension "d17" = 15
extrude "Extrusion1" add sketch "Esquisse1" along normal blind 20 contours L0 L1 L2 L3 in plane through (0, 0, 25) normal (0, 0, 1) makes body 1
sketch "Esquisse2" plane through (0, 0, 0) normal (-1, 0, 0) x (0, -1, 0)
  line L0 (0, 25) -> (15, 25)
  line L1 (15, 25) -> (15, 45)
  line L2 (15, 45) -> (0, 45)
  line L3 (0, 45) -> (0, 25)
  line L4 (0, 35) -> (8, 35)
  line L5 (8, 35) -> (8, 38)
  line L6 (8, 38) -> (0, 38)
  line L7 (0, 38) -> (0, 35)
  dimension "d20" = 8
  dimension "d21" = 3
  constraint horizontal L4
  constraint vertical L5
  constraint horizontal L6
  constraint vertical L7
  constraint midpoint L3 L4.start
  measures "d20" distance of L4.start L4.end
  measures "d21" distance of L4.start L6.end
extrude "Extrusion2" cut sketch "Esquisse2" against normal blind 8 contours L3 L4 L5 L6 L7 bodies 1
sketch "Esquisse3" plane through (0, 0, 45) normal (0, 0, 1) x (-1, 0, 0)
  line L0 (0, 15) -> (-15, 15)
  line L1 (-15, 15) -> (-15, 0)
  line L2 (-15, 0) -> (0, 0)
  line L3 (0, 0) -> (0, 15)
  circle A0 centre (0, 0) radius 3.5
  dimension "d24" = 7
  constraint coincident L2.end L3.start
  measures "d24" diameter of A0
extrude "Extrusion3" cut sketch "Esquisse3" against normal blind 20 contours L2 L3 A0 picked at (-1.8632, 1.3948) bodies 1
extrude "Extrusion4" cut 1 faces at (6.3148, -3.2974, 35) along direction (0, 0, -1) blind 3 on bodies 1 bodies 1
extrude "Extrusion5" cut 1 faces at (10, -15, 38.3333) along direction (0, 1, 0) blind 3 on bodies 1 bodies 1
extrude "Extrusion6" cut 1 faces at (15, -4, 38.3333) along direction (-1, 0, 0) blind 3 on bodies 1 bodies 1
sketch "Esquisse4" plane through (0, 0, 0) normal (-1, 0, 0) x (0, -1, 0)
  line L0 (12, 25) -> (12, 45)
  line L1 (12, 45) -> (3.5, 45)
  line L2 (3.5, 45) -> (3.5, 38)
  line L3 (3.5, 38) -> (8, 38)
  line L4 (8, 38) -> (8, 32)
  line L5 (8, 32) -> (3.5, 32)
  line L6 (3.5, 32) -> (3.5, 25)
  line L7 (3.5, 25) -> (12, 25)
  circle A0 centre (7.75, 41.5) radius 2
  circle A1 centre (7.75, 28.5) radius 2
  dimension "d33" = 4
  dimension "d34" = 4
  measures "d33" diameter of A0
  measures "d34" diameter of A1
extrude "Extrusion7" cut sketch "Esquisse4" against normal blind 6 contours A0 | A1 bodies 1
sketch "Esquisse5" plane through (0, 0, 0) normal (0, 1, 0) x (-1, 0, 0)
  line L0 (-12, 45) -> (-12, 25)
  line L1 (-12, 25) -> (-3.5, 25)
  line L2 (-3.5, 25) -> (-3.5, 32)
  line L3 (-3.5, 32) -> (-8, 32)
  line L4 (-8, 32) -> (-8, 38)
  line L5 (-8, 38) -> (-3.5, 38)
  line L6 (-3.5, 38) -> (-3.5, 45)
  line L7 (-3.5, 45) -> (-12, 45)
  circle A0 centre (-7.75, 41.5) radius 1.75
  circle A1 centre (-7.75, 28.5) radius 1.75
  dimension "d37" = 3.5
  dimension "d38" = 3.5
  measures "d37" diameter of A0
  measures "d38" diameter of A1
extrude "Extrusion8" add sketch "Esquisse5" along normal blind 4 contours A0 | A1 bodies 1
extrude "Extrusion9" add 2 faces at (6, -7.5064, 28.7863) (6, -7.1494, 41.2107) along direction (-1, 0, 0) blind 1 on bodies 1 bodies 1
sketch "Esquisse6" plane through (0, 0, 0) normal (0, 1, 0) x (-1, 0, 0)
  circle A0 centre (-7.75, 28.5) radius 1.75
  circle A1 centre (-7.75, 41.5) radius 1.75
  line L0 (-12, 45) -> (-12, 25)
  line L1 (-12, 25) -> (-3.5, 25)
  line L2 (-3.5, 25) -> (-3.5, 32)
  line L3 (-3.5, 32) -> (-8, 32)
  line L4 (-8, 32) -> (-8, 38)
  line L5 (-8, 38) -> (-3.5, 38)
  line L6 (-3.5, 38) -> (-3.5, 45)
  line L7 (-3.5, 45) -> (-12, 45)
  line L8 (-12, 45) -> (-24, 45)
  line L9 (-24, 45) -> (-24, 25)
  line L10 (-24, 25) -> (-12, 25)
  line L11 (-12, 25) -> (-12, 45)
  line L12 (-24, 40) -> (-14, 40)
  line L13 (-14, 40) -> (-14, 30)
  line L14 (-14, 30) -> (-24, 30)
  line L15 (-24, 30) -> (-24, 40)
  circle A2 centre (-19, 35) radius 2
  line L16 (-14, 40) -> (-12, 40)
  line L17 (-12, 40) -> (-12, 30)
  line L18 (-12, 30) -> (-14, 30)
  line L19 (-14, 30) -> (-14, 40)
  dimension "d43" = 12
  dimension "d44" = 10
  dimension "d45" = 4
  constraint horizontal L8
  constraint vertical L9
  constraint horizontal L10
  constraint vertical L11
  constraint coincident L0.start L7.end
  constraint horizontal L12
  constraint vertical L13
  constraint horizontal L14
  constraint vertical L15
  constraint coincident L9 L12.start
  constraint horizontal L16
  constraint vertical L17
  constraint horizontal L18
  constraint vertical L19
  constraint coincident L11 L17.end
  measures "d43" distance of L0.start L8.end
  measures "d44" distance of L12.start L12.end
  measures "d45" diameter of A2
extrude "Extrusion10" add sketch "Esquisse6" against normal blind 10 contours L0 L11 L13 L16 L17 L18 L19 | L9 L12 L13 L14 L15 L19 bodies 1
extrude "Extrusion11" cut sketch "Esquisse6" against normal blind 6 contours L0 L11 L13 L16 L17 L18 L19 | L9 L12 L13 L14 L15 L19 bodies 1
sketch "Esquisse7" plane through (0, 0, 0) normal (-1, 0, 0) x (0, -1, 0)
  circle A0 centre (7.75, 41.5) radius 2
  circle A1 centre (7.75, 28.5) radius 2
  line L0 (12, 25) -> (12, 45)
  line L1 (12, 45) -> (3.5, 45)
  line L2 (3.5, 45) -> (3.5, 38)
  line L3 (3.5, 38) -> (8, 38)
  line L4 (8, 38) -> (8, 32)
  line L5 (8, 32) -> (3.5, 32)
  line L6 (3.5, 32) -> (3.5, 25)
  line L7 (3.5, 25) -> (12, 25)
  line L8 (12, 45) -> (24, 45)
  line L9 (24, 45) -> (24, 25)
  line L10 (24, 25) -> (12, 25)
  line L11 (12, 25) -> (12, 45)
  line L12 (24, 40) -> (14, 40)
  line L13 (14, 40) -> (14, 30)
  line L14 (14, 30) -> (24, 30)
  line L15 (24, 30) -> (24, 40)
  line L16 (14, 40) -> (12, 40)
  line L17 (12, 40) -> (12, 30)
  line L18 (12, 30) -> (14, 30)
  line L19 (14, 30) -> (14, 40)
  circle A2 centre (19, 35) radius 2
  dimension "d50" = 12
  dimension "d51" = 10
  dimension "d52" = 10
  dimension "d53" = 4
  constraint horizontal L8
  constraint vertical L9
  constraint horizontal L10
  constraint vertical L11
  constraint coincident L0.end L1.start
  constraint horizontal L12
  constraint vertical L13
  constraint horizontal L14
  constraint vertical L15
  constraint horizontal L16
  constraint vertical L17
  constraint horizontal L18
  constraint vertical L19
  constraint coincident L11 L17.end
  measures "d50" distance of L0.end L8.end
  measures "d51" distance of L12.start L12.end
  measures "d52" distance of L12.start L14.end
  measures "d53" diameter of A2
extrude "Extrusion12" add sketch "Esquisse7" against normal blind 10 contours L0 L11 L13 L16 L17 L18 L19 | L9 L12 L13 L14 L15 L19 bodies 1
extrude "Extrusion13" cut sketch "Esquisse7" against normal blind 6 contours L0 L11 L13 L16 L17 L18 L19 | L9 L12 L13 L14 L15 L19 bodies 1
sketch "Esquisse8" plane through (0, 0, 30) normal (0, 0, -1) x (1, 0, 0)
  line L0 (12, 6) -> (24, 6)
  line L1 (24, 6) -> (24, 10)
  line L2 (24, 10) -> (12, 10)
  line L3 (12, 10) -> (12, 6)
  line L4 (10, 24) -> (24, 24)
  line L5 (24, 24) -> (24, 10)
  line L6 (24, 10) -> (10, 10)
  line L7 (10, 10) -> (10, 24)
  circle A0 centre (24, 24) radius 14
  point P0 (10, 24)
  constraint horizontal L4
  constraint vertical L5
  constraint horizontal L6
  constraint vertical L7
  constraint coincident L1.end L2.start
  constraint coincident P0 L4.start
  constraint coincident L4.end L5.start
  constraint coincident L1.end A0
extrude "Extrusion14" add sketch "Esquisse8" against normal blind 10 contours L2 L6 L7 A0 bodies 1
extrude "Extrusion15" cut 1 faces at (19.4157, -10, 35.5212) along direction (0, 1, 0) up to surface end surface at (23.3339, -10.0159, 36.6667) on bodies 1 bodies 1
extrude "Extrusion16" cut 1 faces at (10, -19.5583, 34.7238) along direction (-1, 0, 0) up to surface end surface at (22.9927, -10.0363, 35.0226) on bodies 1 bodies 1
sketch "Esquisse9" plane through (12, 0, 0) normal (1, 0, 0) x (0, 1, 0)
  line L0 (-6, 30) -> (-12, 30)
  line L1 (-12, 30) -> (-12, 25)
  line L2 (-12, 25) -> (0, 25)
  line L3 (0, 25) -> (0, 45)
  line L4 (0, 45) -> (-12, 45)
  line L5 (-12, 45) -> (-12, 40)
  line L6 (-12, 40) -> (-6, 40)
  line L7 (-6, 40) -> (-6, 30)
  line L8 (-6, 45) -> (-4, 45)
  line L9 (-4, 45) -> (-4, 43)
  line L10 (-4, 43) -> (-6, 43)
  line L11 (-6, 43) -> (-6, 45)
  line L12 (-6, 43) -> (-6, 45)
  line L13 (-6, 45) -> (-8, 45)
  line L14 (-8, 43) -> (-6, 43)
  line L15 (-8, 45) -> (-8, 43)
  dimension "d64" = 2
  dimension "d65" = 2
  constraint horizontal L8
  constraint vertical L9
  constraint horizontal L10
  constraint vertical L11
  constraint midpoint L4 L8.start
  constraint symmetric L8.start L11 L12.end
  constraint symmetric L8.end L11 L13.end
  constraint symmetric L9.end L11 L14.start
  constraint symmetric L10.end L11 L12.start
  measures "d64" distance of L8.start L8.end
  measures "d65" distance of L8.start L10.end
extrude "Extrusion17" add sketch "Esquisse9" along normal blind 1 contours L4 L11 L12 L13 L14 L15 | L4 L8 L9 L10 L11 L12 bodies 1
sketch "Esquisse10" plane through (0, -4, 0) normal (0, 1, 0) x (-1, 0, 0)
  line L0 (-12, 43) -> (-12, 45)
  line L1 (-12, 45) -> (-13, 45)
  line L2 (-13, 45) -> (-13, 43)
  line L3 (-13, 43) -> (-12, 43)
  line L4 (-13, 43) -> (-12, 45)
  constraint coincident L2.end L3.start
  constraint coincident L0.end L1.start
extrude "Extrusion18" cut sketch "Esquisse10" against normal blind 4 contours L1 L2 L4 bodies 1
sketch "Esquisse11" plane through (12, 0, 0) normal (1, 0, 0) x (0, 1, 0)
  line L0 (-8, 43) -> (-8, 45)
  line L1 (-8, 45) -> (-12, 45)
  line L2 (-12, 45) -> (-12, 40)
  line L3 (-12, 40) -> (-6, 40)
  line L4 (-6, 40) -> (-6, 30)
  line L5 (-6, 30) -> (-12, 30)
  line L6 (-12, 30) -> (-12, 25)
  line L7 (-12, 25) -> (0, 25)
  line L8 (0, 25) -> (0, 45)
  line L9 (0, 45) -> (-4, 45)
  line L10 (-4, 45) -> (-4, 43)
  line L11 (-4, 43) -> (-8, 43)
sketch "Esquisse12" plane through (0, -12, 0) normal (0, -1, 0) x (1, 0, 0)
  line L0 (12, 30) -> (6, 30)
  line L1 (6, 30) -> (6, 40)
  line L2 (6, 40) -> (12, 40)
  line L3 (12, 40) -> (12, 45)
  line L4 (12, 45) -> (0, 45)
  line L5 (0, 45) -> (0, 25)
  line L6 (0, 25) -> (12, 25)
  line L7 (12, 25) -> (12, 30)
  line L8 (6, 25) -> (8, 25)
  line L9 (8, 25) -> (8, 27)
  line L10 (8, 27) -> (6, 27)
  line L11 (6, 27) -> (6, 25)
  line L12 (6, 27) -> (6, 25)
  line L13 (6, 25) -> (4, 25)
  line L14 (4, 27) -> (6, 27)
  line L15 (4, 25) -> (4, 27)
  dimension "d70" = 2
  dimension "d71" = 2
  constraint horizontal L8
  constraint vertical L9
  constraint horizontal L10
  constraint vertical L11
  constraint midpoint L6 L8.start
  constraint symmetric L8.start L11 L12.end
  constraint symmetric L8.end L11 L13.end
  constraint symmetric L9.end L11 L14.start
  constraint symmetric L10.end L11 L12.start
  measures "d70" distance of L8.start L8.end
  measures "d71" distance of L8.start L10.end
extrude "Extrusion19" add sketch "Esquisse12" along normal blind 1 contours L6 L8 L9 L10 L11 L12 | L6 L11 L12 L13 L14 L15 bodies 1
sketch "Esquisse13" plane through (4, 0, 0) normal (-1, 0, 0) x (0, -1, 0)
  line L0 (12, 27) -> (12, 25)
  line L1 (12, 25) -> (13, 25)
  line L2 (13, 25) -> (13, 27)
  line L3 (13, 27) -> (12, 27)
  line L4 (12, 25) -> (12.1, 25.2)
  line L5 (12.1, 25.2) -> (13, 27)
  constraint coincident L0.end L1.start
  constraint coincident L2.end L3.start
extrude "Extrusion20" cut sketch "Esquisse13" against normal blind 4 contours L1 L2 L4 L5 bodies 1
extrude "Extrusion21" cut 1 faces at (12.3333, -4, 43.6667) along direction (0, -1, 0) blind 4 on bodies 1 bodies 1
extrude "Extrusion22" add 2 faces at (5, -7.1494, 41.2107) (5, -7.5064, 28.7863) along direction (-1, 0, 0) blind 5 on bodies 1 bodies 1
extrude "Extrusion23" cut 2 faces at (7.8798, 4, 42.0687) (8.0417, 4, 29.0052) along direction (0, -1, 0) blind 4 on bodies 1 bodies 1
extrude "Extrusion24" cut 1 faces at (4, -12.3667, 26.4) along direction (1, 0, 0) blind 4 on bodies 1 bodies 1
extrude "Extrusion25" add 1 faces at (6.3148, -3.2974, 38) along direction (0, 0, -1) blind 6 on bodies 1 bodies 1
pattern_circular "Réseau C1" count 4 over 360 about axis through (0, 0, 1.75) along (0, 0, 1) of bodies 1 makes body 2 at (10.0363, 22.9927, 35.0226) makes body 3 at (-22.9927, 10.0363, 35.0226) makes body 4 at (-10.0363, -22.9927, 35.0226)